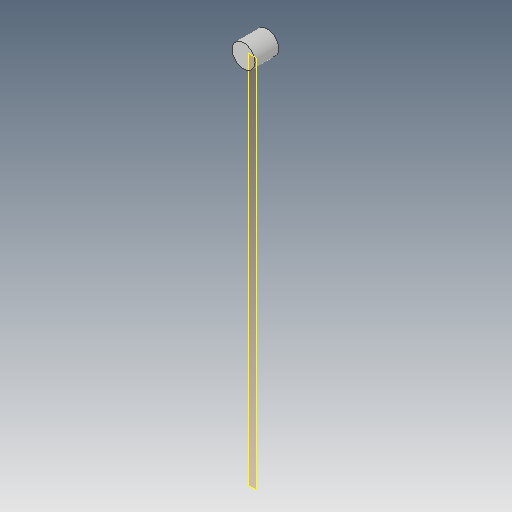
# Autodesk Inventor part: Neje_Gear_End
Saved by Autodesk Inventor 2019.4 (Build 234330000, 330)
## iProperties
Created: 2021-04-08
Part Number: Neje_Gear_End
Material: Generic
Document SubType Name: Modeling
Designer: diederichbenedict
Density: 1 g/cm^3
Appearance: Default
Author: diederichbenedict
Autodesk Inventor part; units mm, degrees
ref_plane "YZ Plane" through (0, 0, 0) normal (1, 0, 0) x (0, 1, 0)
ref_plane "XZ Plane" through (0, 0, 0) normal (0, 1, 0) x (-1, 0, 0)
ref_plane "Work Plane1" through (0, 0, 0) normal (0, 0, 1) x (1, 0, 0)
sketch "Sketch1" plane through (0, 0, 0) normal (0, 0, 1) x (1, 0, 0)
  line L0 (10.525, 153) -> (10.525, -60) projected
  line L1 (14.9, -60) -> (10.525, -60) projected
  line L2 (14.9, 153) -> (14.9, -60) projected
  line L3 (10.525, 153) -> (14.9, 153) projected
  line L4 (4.375, -60) -> (4.375, 153) projected
  line L5 (0, 153) -> (4.375, 153) projected
  line L6 (0, 153) -> (0, -60) projected
  line L7 (4.375, -60) -> (0, -60) projected
  circle A0 centre (7.2233, 160.7618) radius 7.2235
  point P0 (0, 0)
  constraints: 1 centre point
ref_plane "Work Plane2" through (0, -60, -14.9) normal (0, 0, -1) x (0, 1, 0)
extrude "Extrusion1" add sketch "Sketch1" against normal up to surface (14.9 mm away) contours A0
body "Solid1"
